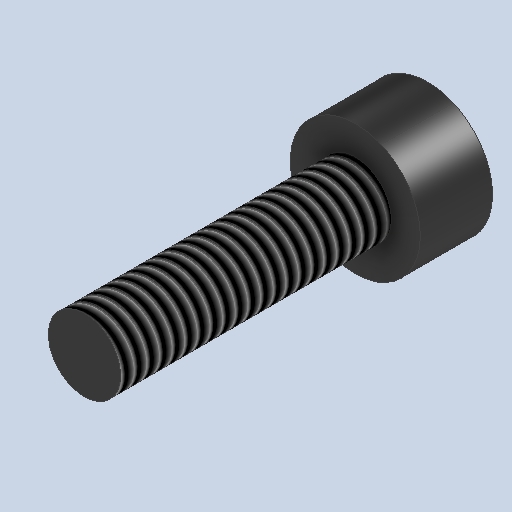
# Autodesk Inventor part: Bolt_M3_15_for_SetCollar_d6
Saved by Autodesk Inventor 2023 (Build 270158000, 158)
## iProperties
Created: 2020-10-10
Part Number: Bolt_M3_15_for_SetCollar_d6
Material: ステンレス鋼
Document SubType Name: Modeling
Designer: yuta2
Density: 8 g/cm^3
Appearance: 光沢 - 黒
Author: yuta2
Autodesk Inventor part; units mm, degrees
ref_plane "YZ Plane" through (0, 0, 0) normal (1, 0, 0) x (0, 1, 0)
ref_plane "XZ Plane" through (0, 0, 0) normal (0, 1, 0) x (-1, 0, 0)
ref_plane "XY Plane" through (0, 0, 0) normal (0, 0, 1) x (1, 0, 0)
sketch "スケッチ1" plane through (0, 0, 0) normal (0, 0, 1) x (1, 0, 0)
  circle A0 centre (0, 0) radius 3.6
  dimension "d0" = 7.2
  constraints: 1 centre point, 1 coincident
  measures "d0" diameter of A0
extrude "押し出し1" add sketch "スケッチ1" along normal blind 4
sketch "スケッチ2" plane through (0, 0, 4) normal (0, 0, 1) x (1, 0, 0)
  circle A0 centre (0, 0) radius 2
  dimension "d3" = 4
  constraints: 1 centre point, 1 coincident
  measures "d3" diameter of A0
extrude "押し出し2" add sketch "スケッチ2" along normal blind 15
thread "ねじ1" size "M4x0.7" class "6g" standard "ISO Metric profile" full length
sketch "スケッチ3" plane through (0, 0, 0) normal (0, 0, -1) x (-1, 0, 0)
  line L0 (0, -2.0207) -> (-1.75, -1.0104)
  line L1 (-1.75, -1.0104) -> (-1.75, 1.0104)
  line L2 (-1.75, 1.0104) -> (0, 2.0207)
  line L3 (0, 2.0207) -> (1.75, 1.0104)
  line L4 (1.75, 1.0104) -> (1.75, -1.0104)
  line L5 (1.75, -1.0104) -> (0, -2.0207)
  point P0 (0, 0)
  point P1 (0, 0)
  dimension "d8" = 3.5
  constraints: 12 end point, 1 coincident, 1 vertical alignment, 13 other
  measures "d8" distance between parallel lines of L1 L4
extrude "押し出し3" cut sketch "スケッチ3" against normal blind 2
